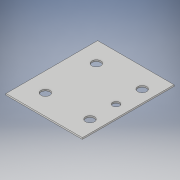
# Autodesk Inventor part: Fixação caixa-tubo
Saved by Autodesk Inventor 2019.4 (Build 234330000, 330)
## iProperties
Created: 2021-05-17
Part Number: Fixação caixa-tubo
Material: Genérico
Document SubType Name: Modeling
Designer: Lattes
Density: 1 g/cm^3
Appearance: Padrão
Author: Lattes
Autodesk Inventor part; units mm, degrees
ref_plane "YZ Plane" through (0, 0, 0) normal (1, 0, 0) x (0, 1, 0)
ref_plane "XZ Plane" through (0, 0, 0) normal (0, 1, 0) x (-1, 0, 0)
ref_plane "XY Plane" through (0, 0, 0) normal (0, 0, 1) x (1, 0, 0)
sketch "Esboço2" plane through (0, 0, 0) normal (0, 1, 0) x (-1, 0, 0)
  line L0 (0, 0) -> (60, 0)
  line L1 (60, 0) -> (60, -12)
  line L2 (60, -12) -> (60, -19)
  line L3 (60, -19) -> (60, -53)
  line L4 (60, -53) -> (60, -60)
  line L5 (60, -60) -> (60, -72)
  line L6 (60, -72) -> (0, -72)
  line L7 (0, -72) -> (0, 0)
  line L8 (0, 0) -> (19, 0)
  line L9 (60, 0) -> (30, 0)
  circle A0 centre (45, -16) radius 3.5
  circle A1 centre (45, -56) radius 3.5
  circle A2 centre (9.5, -15.5) radius 3.5
  circle A3 centre (9.5, -56.5) radius 3.5
  circle A4 centre (9.5, -36) radius 2.7
  dimension "d13" = 60
  dimension "d14" = 12
  dimension "d15" = 7
  dimension "d16" = 34
  dimension "d17" = 7
  dimension "d18" = 12
  dimension "d19" = 72
  dimension "d20" = 19
  dimension "d21" = 30
  dimension "d22" = 7
  dimension "d23" = 7
  dimension "d24" = 7
  dimension "d25" = 7
  constraints: 20 end point, 5 centre point, 4 point on line, 3 perpendicular, 1 horizontal, 1 midpoint, 1 vertical
  measures "d13" distance of L0.start L0.end
  measures "d14" distance of L0.end L1.end
  measures "d15" distance of L1.end L2.end
  measures "d16" distance of L2.end L3.end
  measures "d17" distance of L3.end L4.end
  measures "d18" distance of L4.end L5.end
  measures "d19" distance of L6.end L0.start
  measures "d20" distance of L0.start L8.end
  measures "d21" distance of L0.end L9.end
  measures "d22" diameter of A0
  measures "d23" diameter of A1
  measures "d24" diameter of A2
  measures "d25" diameter of A3
extrude "Extrusão1" add sketch "Esboço2" along normal blind 1.2
